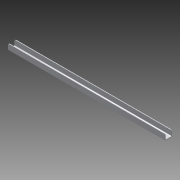
# Autodesk Inventor part: alignmentWheelsBar
Saved by Autodesk Inventor 2015 (Build 190159000, 159)
## iProperties
Created: 2015-01-30
Part Number: alignmentWheelsBar
Material: Generic
Document SubType Name: Modeling
Designer: Kingbob26
Density: 1 g/cm^3
Appearance: Default
Author: Kingbob26
Autodesk Inventor part; units mm, degrees
ref_plane "YZ Plane" through (0, 0, 0) normal (1, 0, 0) x (0, 1, 0)
ref_plane "XZ Plane" through (0, 0, 0) normal (0, 1, 0) x (-1, 0, 0)
ref_plane "XY Plane" through (0, 0, 0) normal (0, 0, 1) x (1, 0, 0)
sketch "Sketch1" plane through (0, 0, 0) normal (0, 1, 0) x (-1, 0, 0)
  point P0 (0, 0)
sketch "Sketch2" plane through (0, 0, 0) normal (0, 1, 0) x (-1, 0, 0)
  line L0 (381, 15.875) -> (-381, 15.875)
  line L1 (-381, 15.875) -> (-381, -15.875)
  line L2 (-381, -15.875) -> (381, -15.875)
  line L3 (381, -15.875) -> (381, 15.875)
  point P0 (0, 0)
  dimension "d2" = 762
  dimension "d3" = 31.75
  constraints: 8 end point, 2 parallel, 1 horizontal, 1 perpendicular
  measures "d2" distance of L2.end L1.end
  measures "d3" distance of L1.end L0.end
extrude "Extrusion1" add sketch "Sketch2" along normal blind 3.175
sketch "Sketch3" plane through (381, 0, -15.875) normal (0, 0, -1) x (-1, 0, 0)
  point P0 (381, 0)
sketch "Sketch4" plane through (0, 0, 0) normal (0, -1, 0) x (1, 0, 0)
  point P0 (0, 0)
sketch "Sketch5" plane through (0, 0, 0) normal (0, -1, 0) x (1, 0, 0)
  line L0 (381, -15.875) -> (-381, -15.875)
  line L1 (-381, -15.875) -> (-381, -19.05)
  line L2 (-381, -19.05) -> (381, -19.05)
  line L3 (381, -19.05) -> (381, -15.875)
  point P0 (0, 0)
  dimension "d6" = 762
  dimension "d7" = 3.175
  constraints: 8 end point, 2 parallel, 1 horizontal, 1 perpendicular
  measures "d6" distance of L2.end L1.end
  measures "d7" distance of L1.end L0.end
extrude "Extrusion2" add sketch "Sketch5" against normal blind 3.175
sketch "Sketch6" plane through (-381, 0, 15.875) normal (0, 0, 1) x (1, 0, 0)
  line L0 (0, 0) -> (762, 0)
  line L1 (762, 0) -> (762, 28.575)
  line L2 (762, 28.575) -> (0, 28.575)
  line L3 (0, 28.575) -> (0, 0)
  point P0 (381, 0)
  dimension "d10" = 762
  dimension "d11" = 28.575
  constraints: 8 end point, 2 parallel, 1 horizontal, 1 perpendicular
  measures "d10" distance of L2.end L1.end
  measures "d11" distance of L1.end L0.end
sketch "Sketch7" plane through (0, 3.175, 0) normal (0, 1, 0) x (1, 0, 0)
  line L0 (-381, -15.875) -> (381, -15.875)
  line L1 (381, -15.875) -> (381, -12.7)
  line L2 (381, -12.7) -> (-381, -12.7)
  line L3 (-381, -12.7) -> (-381, -15.875)
  point P0 (0, 0)
  dimension "d12" = 762
  dimension "d13" = 3.175
  constraints: 8 end point, 2 parallel, 1 horizontal, 1 perpendicular
  measures "d12" distance of L2.end L1.end
  measures "d13" distance of L1.end L0.end
extrude "Extrusion3" cut sketch "Sketch7" against normal blind 3.175
extrude "Extrusion4" add sketch "Sketch6" against normal blind 3.175
sketch "Sketch8" plane through (0, 3.175, 0) normal (0, 1, 0) x (1, 0, 0)
  point P0 (0, 0)
sketch "Sketch9" plane through (381, 0, -19.05) normal (0, 0, -1) x (-1, 0, 0)
  line L0 (0, 0) -> (762, 0)
  line L1 (762, 0) -> (762, 28.575)
  line L2 (762, 28.575) -> (0, 28.575)
  line L3 (0, 28.575) -> (0, 0)
  point P0 (381, 0)
  dimension "d18" = 762
  dimension "d19" = 28.575
  constraints: 8 end point, 2 parallel, 1 horizontal, 1 perpendicular
  measures "d18" distance of L2.end L1.end
  measures "d19" distance of L1.end L0.end
sketch "Sketch10" plane through (0, 3.175, 0) normal (0, 1, 0) x (1, 0, 0)
  line L0 (381, 19.05) -> (-381, 19.05)
  line L1 (-381, 19.05) -> (-381, 15.875)
  line L2 (-381, 15.875) -> (381, 15.875)
  line L3 (381, 15.875) -> (381, 19.05)
  point P0 (0, 0)
  dimension "d20" = 762
  dimension "d21" = 3.175
  constraints: 8 end point, 2 parallel, 1 horizontal, 1 perpendicular
  measures "d20" distance of L2.end L1.end
  measures "d21" distance of L1.end L0.end
extrude "Extrusion5" cut sketch "Sketch10" against normal blind 3.175
extrude "Extrusion6" add sketch "Sketch9" against normal blind 3.175
fillet "Fillet1" radius 3.175 1 edges at (0, 3.175, 12.7)
fillet "Fillet2" radius 3.175 1 edges at (0, 3.175, -15.875)
fillet "Fillet3" radius 3.175 1 edges at (0, 0, 15.875)
fillet "Fillet4" radius 3.175 1 edges at (0, 0, -19.05)
fillet "Fillet5" radius 6.35 1 edges at (-381, 28.575, -17.4625)
fillet "Fillet6" radius 6.35 1 edges at (-381, 28.575, 14.2875)
fillet "Fillet7" radius 6.35 1 edges at (381, 28.575, 14.2875)
fillet "Fillet8" radius 6.35 1 edges at (381, 28.575, -17.4625)
body "Solid1"
